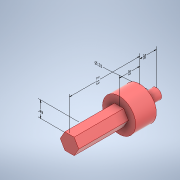
# Autodesk Inventor part: 1x8mmx1_5-inchHexShaft
Saved by Autodesk Inventor 2022.1 (Build 261234000, 234)
## iProperties
Created: 2020-11-16
Part Number: 1x8mmx1_5-inchHexShaft
Material: PC/ABS Plastic
Document SubType Name: Modeling
Designer: robst
Density: 0.357273 g/cm^3
Appearance: Smooth - Red
Author: robst
Autodesk Inventor part; units mm, degrees
ref_plane "YZ Plane" through (0, 0, 0) normal (1, 0, 0) x (0, 1, 0)
ref_plane "XZ Plane" through (0, 0, 0) normal (0, 1, 0) x (-1, 0, 0)
ref_plane "XY Plane" through (0, 0, 0) normal (0, 0, 1) x (1, 0, 0)
sketch "Sketch1" plane through (0, 0, 0) normal (0, 0, 1) x (1, 0, 0)
  line L0 (7.3323, 0) -> (3.6662, -6.35)
  line L1 (3.6662, -6.35) -> (-3.6662, -6.35)
  line L2 (-3.6662, -6.35) -> (-7.3323, 0)
  line L3 (-7.3323, 0) -> (-3.6662, 6.35)
  line L4 (-3.6662, 6.35) -> (3.6662, 6.35)
  line L5 (3.6662, 6.35) -> (7.3323, 0)
  point P0 (0, 0)
  point P1 (0, 0)
  dimension "d0" = 12.7
  constraints: 12 end point, 1 coincident, 1 horizontal, 13 other
  measures "d0" distance between parallel lines of L1 L4
extrude "Extrusion1" add sketch "Sketch1" along normal mid plane 38.1
sketch "Sketch2" plane through (0, 0, -19.05) normal (0, 0, -1) x (-1, 0, 0)
  circle A0 centre (0, 0) radius 12.7
  dimension "d3" = 25.4
  constraints: 1 centre point, 1 coincident
  measures "d3" diameter of A0
extrude "Extrusion2" add sketch "Sketch2" along normal blind 15.875
thicken "Reduce Size of Hex Shaft" operation add thickness 0.1905 both sides no extend neighbours yes toward (-0.8660254, -0.5, 0) faces at (6.1103, 2.1167, -6.35) (-1.2221, 6.35, 6.35) (4.8882, -4.2333, -6.35) (-1.2221, -6.35, -6.35) (-4.8882, -4.2333, 6.35) (-6.1103, 2.1167, 6.35)
sketch "Sketch3" plane through (0, 0, -34.925) normal (0, 0, -1) x (-1, 0, 0)
  circle A0 centre (0, 0) radius 4
  dimension "d14" = 8
  constraints: 1 centre point, 1 coincident
  measures "d14" diameter of A0
extrude "Extrusion3" add sketch "Sketch3" along normal blind 12.7
equation "\"d0\" = hexSize"
equation "\"d1\" = length"
equation "\"d6\" = printOffset"
equation "\"hexSize\" = 12.7"
equation "\"length\" = 38.1"
equation "\"printOffset\" = 0.1905"
body "Solid1"
